Autodesk Fusion 360 part; units mm, degrees
(part 17 of 18)
  spline S9 degree 5 poles (6.448875, 0.349392) (6.446894, 0.350948) (6.442931, 0.354057) (6.436987, 0.358705) (6.429063, 0.364874) (6.419158, 0.372539) (6.409254, 0.380155) (6.399351, 0.387725) (6.389449, 0.395247) (6.379548, 0.402722) (6.369649, 0.410149) (6.359751, 0.417529) (6.349856, 0.424862) (6.339962, 0.432147) (6.330071, 0.439384) (6.320183, 0.446575) (6.310298, 0.453717) (6.300416, 0.460813) (6.290538, 0.467861) (6.280664, 0.474861) (6.270793, 0.481815) (6.260927, 0.48872) (6.251065, 0.495579) (6.241208, 0.50239) (6.231356, 0.509153) (6.221509, 0.515869) (6.211668, 0.522538) (6.201832, 0.52916) (6.192002, 0.535734) (6.182179, 0.54226) (6.172362, 0.54874) (6.162551, 0.555172) (6.152748, 0.561557) (6.142952, 0.567894) (6.133163, 0.574185) (6.123382, 0.580428) (6.113609, 0.586623) (6.103844, 0.592772) (6.094088, 0.598873) (6.084341, 0.604928) (6.074602, 0.610935) (6.064873, 0.616895) (6.055154, 0.622808) (6.045444, 0.628674) (6.035744, 0.634492) (6.026055, 0.640264) (6.016376, 0.645989) (6.006708, 0.651667) (5.997052, 0.657298) (5.987406, 0.662882) (5.977773, 0.66842) (5.968151, 0.67391) (5.958542, 0.679354) (5.948945, 0.684751) (5.93936, 0.690101) (5.929789, 0.695405) (5.920232, 0.700662) (5.910687, 0.705873) (5.901157, 0.711037) (5.891641, 0.716155) (5.882139, 0.721226) (5.872652, 0.726251) (5.86318, 0.73123) (5.853723, 0.736162) (5.844282, 0.741048) (5.834857, 0.745888) (5.825447, 0.750682) (5.816054, 0.75543) (5.806678, 0.760132) (5.797319, 0.764788) (5.787977, 0.769398) (5.778653, 0.773962) (5.769346, 0.778481) (5.760058, 0.782954) (5.750788, 0.787381) (5.741537, 0.791763) (5.732305, 0.7961) (5.723092, 0.800391) (5.713899, 0.804636) (5.704726, 0.808837) (5.695573, 0.812992) (5.686441, 0.817103) (5.677329, 0.821168) (5.668238, 0.825188) (5.659169, 0.829164) (5.650122, 0.833095) (5.641097, 0.836981) (5.632094, 0.840823) (5.623114, 0.84462) (5.614157, 0.848373) (5.605223, 0.852081) (5.596312, 0.855745) (5.587426, 0.859365) (5.578564, 0.862942) (5.569726, 0.866474) (5.560914, 0.869962) (5.552126, 0.873407) (5.543364, 0.876808) (5.534628, 0.880166) (5.525918, 0.88348) (5.517235, 0.886752) (5.508578, 0.88998) (5.499949, 0.893164) (5.491347, 0.896307) (5.482773, 0.899406) (5.474226, 0.902462) (5.465709, 0.905476) (5.45722, 0.908448) (5.448761, 0.911377) (5.44033, 0.914264) (5.43193, 0.917109) (5.42356, 0.919913) (5.41522, 0.922674) (5.406911, 0.925394) (5.398634, 0.928072) (5.390388, 0.930709) (5.382174, 0.933305) (5.373992, 0.93586) (5.365842, 0.938374) (5.357726, 0.940847) (5.349643, 0.943279) (5.341593, 0.945672) (5.333578, 0.948023) (5.325597, 0.950335) (5.317651, 0.952607) (5.30974, 0.954839) (5.301864, 0.957031) (5.294024, 0.959184) (5.28622, 0.961298) (5.278453, 0.963372) (5.270723, 0.965408) (5.263031, 0.967405) (5.255375, 0.969364) (5.247758, 0.971284) (5.24018, 0.973166) (5.23264, 0.97501) (5.22514, 0.976816) (5.217679, 0.978584) (5.210258, 0.980316) (5.202878, 0.98201) (5.195538, 0.983667) (5.18824, 0.985287) (5.180983, 0.986871) (5.173768, 0.988419) (5.166596, 0.98993) (5.159466, 0.991406) (5.152379, 0.992846) (5.145336, 0.994251) (5.138338, 0.99562) (5.131383, 0.996955) (5.124474, 0.998254) (5.117609, 0.99952) (5.110791, 1.000751) (5.104018, 1.001948) (5.097292, 1.003112) (5.090613, 1.004242) (5.083981, 1.005339) (5.077397, 1.006403) (5.070862, 1.007435) (5.064375, 1.008434) (5.057937, 1.009401) (5.051549, 1.010337) (5.045211, 1.011241) (5.038924, 1.012114) (5.032687, 1.012955) (5.026502, 1.013767) (5.020368, 1.014548) (5.014287, 1.015299) (5.008259, 1.01602) (5.002284, 1.016712) (4.996363, 1.017375) (4.990496, 1.01801) (4.984684, 1.018616) (4.978927, 1.019194) (4.973225, 1.019744) (4.96758, 1.020267) (4.961991, 1.020763) (4.95646, 1.021233) (4.950986, 1.021676) (4.945571, 1.022094) (4.940214, 1.022486) (4.934916, 1.022853) (4.929678, 1.023195) (4.9245, 1.023513) (4.919383, 1.023807) (4.914327, 1.024078) (4.909334, 1.024325) (4.904402, 1.02455) (4.899534, 1.024753) (4.894729, 1.024934) (4.889988, 1.025093) (4.885311, 1.025232) (4.8807, 1.025351) (4.876155, 1.025449) (4.871676, 1.025528) (4.867264, 1.025588) (4.862919, 1.025629) (4.858642, 1.025653) (4.854434, 1.025658) (4.850296, 1.025647) (4.846227, 1.02562) (4.842229, 1.025576) (4.838302, 1.025517) (4.834447, 1.025444) (4.830665, 1.025356) (4.826955, 1.025254) (4.82332, 1.025139) (4.819758, 1.025012) (4.816272, 1.024872) (4.812862, 1.024722) (4.809528, 1.024561) (4.806271, 1.024389) (4.803092, 1.024208) (4.799992, 1.024019) (4.796971, 1.023821) (4.79403, 1.023616) (4.79117, 1.023404) (4.788391, 1.023186) (4.785695, 1.022963) (4.783081, 1.022736) (4.780552, 1.022504) (4.778107, 1.02227) (4.775748, 1.022033) (4.773475, 1.021795) (4.771289, 1.021556) (4.769192, 1.021318) (4.767183, 1.02108) (4.765263, 1.020844) (4.763435, 1.020612) (4.761697, 1.020383) (4.760053, 1.020158) (4.758501, 1.019939) (4.757044, 1.019727) (4.755682, 1.019523) (4.754417, 1.019326) (4.753248, 1.019139) (4.752177, 1.018962) (4.751206, 1.018798) (4.750336, 1.018647) (4.749568, 1.01851) (4.748903, 1.018389) (4.748453, 1.018304) (4.748162, 1.018248) (4.747988, 1.018213) (4.747907, 1.018197) knots -1 -1 -1 -1 -1 -1 -0.99583333 -0.99166667 -0.9875 -0.98333333 -0.97916667 -0.975 -0.97083333 -0.96666667 -0.9625 -0.95833333 -0.95416667 -0.95 -0.94583333 -0.94166667 -0.9375 -0.93333333 -0.92916667 -0.925 -0.92083333 -0.91666667 -0.9125 -0.90833333 -0.90416667 -0.9 -0.89583333 -0.89166667 -0.8875 -0.88333333 -0.87916667 -0.875 -0.87083333 -0.86666667 -0.8625 -0.85833333 -0.85416667 -0.85 -0.84583333 -0.84166667 -0.8375 -0.83333333 -0.82916667 -0.825 -0.82083333 -0.81666667 -0.8125 -0.80833333 -0.80416667 -0.8 -0.79583333 -0.79166667 -0.7875 -0.78333333 -0.77916667 -0.775 -0.77083333 -0.76666667 -0.7625 -0.75833333 -0.75416667 -0.75 -0.74583333 -0.74166667 -0.7375 -0.73333333 -0.72916667 -0.725 -0.72083333 -0.71666667 -0.7125 -0.70833333 -0.70416667 -0.7 -0.69583333 -0.69166667 -0.6875 -0.68333333 -0.67916667 -0.675 -0.67083333 -0.66666667 -0.6625 -0.65833333 -0.65416667 -0.65 -0.64583333 -0.64166667 -0.6375 -0.63333333 -0.62916667 -0.625 -0.62083333 -0.61666667 -0.6125 -0.60833333 -0.60416667 -0.6 -0.59583333 -0.59166667 -0.5875 -0.58333333 -0.57916667 -0.575 -0.57083333 -0.56666667 -0.5625 -0.55833333 -0.55416667 -0.55 -0.54583333 -0.54166667 -0.5375 -0.53333333 -0.52916667 -0.525 -0.52083333 -0.51666667 -0.5125 -0.50833333 -0.50416667 -0.5 -0.49583333 -0.49166667 -0.4875 -0.48333333 -0.47916667 -0.475 -0.47083333 -0.46666667 -0.4625 -0.45833333 -0.45416667 -0.45 -0.44583333 -0.44166667 -0.4375 -0.43333333 -0.42916667 -0.425 -0.42083333 -0.41666667 -0.4125 -0.40833333 -0.40416667 -0.4 -0.39583333 -0.39166667 -0.3875 -0.38333333 -0.37916667 -0.375 -0.37083333 -0.36666667 -0.3625 -0.35833333 -0.35416667 -0.35 -0.34583333 -0.34166667 -0.3375 -0.33333333 -0.32916667 -0.325 -0.32083333 -0.31666667 -0.3125 -0.30833333 -0.30416667 -0.3 -0.29583333 -0.29166667 -0.2875 -0.28333333 -0.27916667 -0.275 -0.27083333 -0.26666667 -0.2625 -0.25833333 -0.25416667 -0.25 -0.24583333 -0.24166667 -0.2375 -0.23333333 -0.22916667 -0.225 -0.22083333 -0.21666667 -0.2125 -0.20833333 -0.20416667 -0.2 -0.19583333 -0.19166667 -0.1875 -0.18333333 -0.17916667 -0.175 -0.17083333 -0.16666667 -0.1625 -0.15833333 -0.15416667 -0.15 -0.14583333 -0.14166667 -0.1375 -0.13333333 -0.12916667 -0.125 -0.12083333 -0.11666667 -0.1125 -0.10833333 -0.10416667 -0.1 -0.09583333 -0.09166667 -0.0875 -0.08333333 -0.07916667 -0.075 -0.07083333 -0.06666667 -0.0625 -0.05833333 -0.05416667 -0.05 -0.04583333 -0.04166667 -0.0375 -0.03333333 -0.02916667 -0.025 -0.02083333 -0.01666667 -0.0125 -0.00833333 -0.00416667 0 0 0 0 0 0
  line L18 (4.747907, 1.018197) -> (4.747144, 1.018043)
  line L19 (4.747144, 1.018043) -> (3.473116, 0.744823)
  arc A10 (3.473116, 0.744823) -> (2.982533, 1.929195) centre (0, 0) ccw
  line L20 (2.982533, 1.929195) -> (4.076603, 2.636873)
  line L21 (4.076603, 2.636873) -> (4.077251, 2.637303)
  spline S10 degree 5 poles (4.077251, 2.637303) (4.07732, 2.637349) (4.077467, 2.637448) (4.077713, 2.637613) (4.078091, 2.637872) (4.078647, 2.638256) (4.079287, 2.638703) (4.080009, 2.639211) (4.080812, 2.639782) (4.081694, 2.640414) (4.082653, 2.641108) (4.083687, 2.641864) (4.084794, 2.642682) (4.085975, 2.643562) (4.087226, 2.644505) (4.088548, 2.645509) (4.089938, 2.646575) (4.091396, 2.647704) (4.09292, 2.648895) (4.094508, 2.650147) (4.09616, 2.651462) (4.097875, 2.652839) (4.09965, 2.654277) (4.101486, 2.655778) (4.10338, 2.657341) (4.105333, 2.658966) (4.107341, 2.660653) (4.109406, 2.662402) (4.111524, 2.664213) (4.113697, 2.666085) (4.115921, 2.66802) (4.118197, 2.670016) (4.120524, 2.672074) (4.122899, 2.674194) (4.125323, 2.676376) (4.127795, 2.678619) (4.130313, 2.680924) (4.132877, 2.683291) (4.135485, 2.685719) (4.138137, 2.688209) (4.140832, 2.69076) (4.143569, 2.693372) (4.146347, 2.696046) (4.149165, 2.698781) (4.152023, 2.701577) (4.154919, 2.704435) (4.157854, 2.707354) (4.160825, 2.710333) (4.163832, 2.713374) (4.166875, 2.716475) (4.169953, 2.719637) (4.173064, 2.72286) (4.176209, 2.726144) (4.179385, 2.729488) (4.182594, 2.732893) (4.185834, 2.736358) (4.189103, 2.739884) (4.192402, 2.74347) (4.19573, 2.747116) (4.199087, 2.750822) (4.20247, 2.754588) (4.20588, 2.758415) (4.209317, 2.762301) (4.212779, 2.766246) (4.216265, 2.770252) (4.219776, 2.774317) (4.22331, 2.778442) (4.226867, 2.782626) (4.230446, 2.786869) (4.234047, 2.791172) (4.237669, 2.795533) (4.241312, 2.799954) (4.244974, 2.804434) (4.248655, 2.808972) (4.252355, 2.813569) (4.256073, 2.818225) (4.259809, 2.822939) (4.263561, 2.827712) (4.26733, 2.832543) (4.271115, 2.837432) (4.274915, 2.842379) (4.278729, 2.847385) (4.282558, 2.852448) (4.286401, 2.857569) (4.290256, 2.862747) (4.294125, 2.867983) (4.298005, 2.873277) (4.301897, 2.878627) (4.3058, 2.884035) (4.309713, 2.8895) (4.313637, 2.895022) (4.31757, 2.900601) (4.321513, 2.906237) (4.325463, 2.911929) (4.329422, 2.917678) (4.333389, 2.923482) (4.337363, 2.929344) (4.341344, 2.935261) (4.34533, 2.941234) (4.349323, 2.947263) (4.353321, 2.953348) (4.357324, 2.959489) (4.361331, 2.965685) (4.365343, 2.971936) (4.369358, 2.978243) (4.373376, 2.984604) (4.377397, 2.991021) (4.38142, 2.997493) (4.385445, 3.004019) (4.389471, 3.0106) (4.393499, 3.017235) (4.397527, 3.023924) (4.401555, 3.030668) (4.405583, 3.037466) (4.409611, 3.044318) (4.413637, 3.051223) (4.417663, 3.058182) (4.421686, 3.065195) (4.425707, 3.072261) (4.429726, 3.07938) (4.433742, 3.086552) (4.437754, 3.093777) (4.441763, 3.101056) (4.445768, 3.108386) (4.449768, 3.11577) (4.453764, 3.123205) (4.457754, 3.130693) (4.461739, 3.138233) (4.465718, 3.145825) (4.469691, 3.153469) (4.473657, 3.161164) (4.477616, 3.168911) (4.481568, 3.17671) (4.485512, 3.184559) (4.489449, 3.19246) (4.493377, 3.200412) (4.497297, 3.208415) (4.501207, 3.216468) (4.505108, 3.224571) (4.509, 3.232725) (4.512882, 3.24093) (4.516753, 3.249184) (4.520614, 3.257488) (4.524464, 3.265842) (4.528302, 3.274246) (4.532129, 3.282699) (4.535945, 3.291202) (4.539748, 3.299753) (4.543538, 3.308354) (4.547316, 3.317004) (4.551081, 3.325702) (4.554832, 3.334449) (4.55857, 3.343244) (4.562294, 3.352087) (4.566003, 3.360979) (4.569698, 3.369918) (4.573378, 3.378906) (4.577043, 3.387941) (4.580693, 3.397023) (4.584327, 3.406153) (4.587945, 3.41533) (4.591546, 3.424554) (4.595131, 3.433824) (4.598699, 3.443142) (4.602251, 3.452506) (4.605784, 3.461916) (4.609301, 3.471373) (4.612799, 3.480876) (4.616279, 3.490424) (4.619741, 3.500019) (4.623184, 3.509659) (4.626608, 3.519344) (4.630013, 3.529075) (4.633399, 3.538851) (4.636764, 3.548671) (4.64011, 3.558537) (4.643436, 3.568447) (4.646741, 3.578402) (4.650026, 3.588401) (4.653289, 3.598444) (4.656532, 3.608531) (4.659752, 3.618662) (4.662952, 3.628837) (4.666129, 3.639055) (4.669284, 3.649317) (4.672417, 3.659621) (4.675527, 3.669969) (4.678615, 3.68036) (4.681679, 3.690793) (4.68472, 3.701269) (4.687737, 3.711787) (4.690731, 3.722347) (4.693701, 3.732949) (4.696647, 3.743594) (4.699568, 3.75428) (4.702464, 3.765007) (4.705336, 3.775776) (4.708182, 3.786586) (4.711004, 3.797437) (4.713799, 3.808329) (4.716569, 3.819262) (4.719314, 3.830235) (4.722032, 3.841249) (4.724723, 3.852302) (4.727389, 3.863396) (4.730027, 3.87453) (4.732638, 3.885704) (4.735223, 3.896917) (4.73778, 3.908169) (4.740309, 3.919461) (4.742811, 3.930791) (4.745285, 3.942161) (4.74773, 3.953569) (4.750148, 3.965016) (4.752536, 3.976501) (4.754896, 3.988024) (4.757228, 3.999586) (4.75953, 4.011185) (4.761803, 4.022822) (4.764046, 4.034497) (4.76626, 4.046208) (4.768444, 4.057958) (4.770598, 4.069744) (4.772721, 4.081567) (4.774815, 4.093426) (4.776878, 4.105322) (4.77891, 4.117255) (4.780911, 4.129223) (4.782881, 4.141228) (4.78482, 4.153268) (4.786728, 4.165345) (4.788604, 4.177456) (4.790449, 4.189603) (4.792261, 4.201786) (4.794041, 4.214003) (4.795789, 4.226254) (4.797505, 4.238541) (4.799187, 4.250862) (4.800837, 4.263216) (4.802455, 4.275606) (4.804039, 4.288029) (4.80528, 4.297995) (4.806196, 4.305485) (4.8068, 4.310485) (4.807101, 4.312986) knots 0 0 0 0 0 0 0.00416667 0.00833333 0.0125 0.01666667 0.02083333 0.025 0.02916667 0.03333333 0.0375 0.04166667 0.04583333 0.05 0.05416667 0.05833333 0.0625 0.06666667 0.07083333 0.075 0.07916667 0.08333333 0.0875 0.09166667 0.09583333 0.1 0.10416667 0.10833333 0.1125 0.11666667 0.12083333 0.125 0.12916667 0.13333333 0.1375 0.14166667 0.14583333 0.15 0.15416667 0.15833333 0.1625 0.16666667 0.17083333 0.175 0.17916667 0.18333333 0.1875 0.19166667 0.19583333 0.2 0.20416667 0.20833333 0.2125 0.21666667 0.22083333 0.225 0.22916667 0.23333333 0.2375 0.24166667 0.24583333 0.25 0.25416667 0.25833333 0.2625 0.26666667 0.27083333 0.275 0.27916667 0.28333333 0.2875 0.29166667 0.29583333 0.3 0.30416667 0.30833333 0.3125 0.31666667 0.32083333 0.325 0.32916667 0.33333333 0.3375 0.34166667 0.34583333 0.35 0.35416667 0.35833333 0.3625 0.36666667 0.37083333 0.375 0.37916667 0.38333333 0.3875 0.39166667 0.39583333 0.4 0.40416667 0.40833333 0.4125 0.41666667 0.42083333 0.425 0.42916667 0.43333333 0.4375 0.44166667 0.44583333 0.45 0.45416667 0.45833333 0.4625 0.46666667 0.47083333 0.475 0.47916667 0.48333333 0.4875 0.49166667 0.49583333 0.5 0.50416667 0.50833333 0.5125 0.51666667 0.52083333 0.525 0.52916667 0.53333333 0.5375 0.54166667 0.54583333 0.55 0.55416667 0.55833333 0.5625 0.56666667 0.57083333 0.575 0.57916667 0.58333333 0.5875 0.59166667 0.59583333 0.6 0.60416667 0.60833333 0.6125 0.61666667 0.62083333 0.625 0.62916667 0.63333333 0.6375 0.64166667 0.64583333 0.65 0.65416667 0.65833333 0.6625 0.66666667 0.67083333 0.675 0.67916667 0.68333333 0.6875 0.69166667 0.69583333 0.7 0.70416667 0.70833333 0.7125 0.71666667 0.72083333 0.725 0.72916667 0.73333333 0.7375 0.74166667 0.74583333 0.75 0.75416667 0.75833333 0.7625 0.76666667 0.77083333 0.775 0.77916667 0.78333333 0.7875 0.79166667 0.79583333 0.8 0.80416667 0.80833333 0.8125 0.81666667 0.82083333 0.825 0.82916667 0.83333333 0.8375 0.84166667 0.84583333 0.85 0.85416667 0.85833333 0.8625 0.86666667 0.87083333 0.875 0.87916667 0.88333333 0.8875 0.89166667 0.89583333 0.9 0.90416667 0.90833333 0.9125 0.91666667 0.92083333 0.925 0.92916667 0.93333333 0.9375 0.94166667 0.94583333 0.95 0.95416667 0.95833333 0.9625 0.96666667 0.97083333 0.975 0.97916667 0.98333333 0.9875 0.99166667 0.99583333 1 1 1 1 1 1
  arc A11 (4.807101, 4.312986) -> (4.312986, 4.807101) centre (0, 0) ccw
  spline S11 degree 5 poles (4.312986, 4.807101) (4.310485, 4.8068) (4.305485, 4.806196) (4.297995, 4.80528) (4.288029, 4.804039) (4.275606, 4.802455) (4.263216, 4.800837) (4.250862, 4.799187) (4.238541, 4.797505) (4.226254, 4.795789) (4.214003, 4.794041) (4.201786, 4.792261) (4.189603, 4.790449) (4.177456, 4.788604) (4.165345, 4.786728) (4.153268, 4.78482) (4.141228, 4.782881) (4.129223, 4.780911) (4.117255, 4.77891) (4.105322, 4.776878) (4.093426, 4.774815) (4.081567, 4.772721) (4.069744, 4.770598) (4.057958, 4.768444) (4.046208, 4.76626) (4.034497, 4.764046) (4.022822, 4.761803) (4.011185, 4.75953) (3.999586, 4.757228) (3.988024, 4.754896) (3.976501, 4.752536) (3.965016, 4.750148) (3.953569, 4.74773) (3.942161, 4.745285) (3.930791, 4.742811) (3.919461, 4.740309) (3.908169, 4.73778) (3.896917, 4.735223) (3.885704, 4.732638) (3.87453, 4.730027) (3.863396, 4.727389) (3.852302, 4.724723) (3.841249, 4.722032) (3.830235, 4.719314) (3.819262, 4.716569) (3.808329, 4.713799) (3.797437, 4.711004) (3.786586, 4.708182) (3.775776, 4.705336) (3.765007, 4.702464) (3.75428, 4.699568) (3.743594, 4.696647) (3.732949, 4.693701) (3.722347, 4.690731) (3.711787, 4.687737) (3.701269, 4.68472) (3.690793, 4.681679) (3.68036, 4.678615) (3.669969, 4.675527) (3.659621, 4.672417) (3.649317, 4.669284) (3.639055, 4.666129) (3.628837, 4.662952) (3.618662, 4.659752) (3.608531, 4.656532) (3.598444, 4.653289) (3.588401, 4.650026) (3.578402, 4.646741) (3.568447, 4.643436) (3.558537, 4.64011) (3.548671, 4.636764) (3.538851, 4.633399) (3.529075, 4.630013) (3.519344, 4.626608) (3.509659, 4.623184) (3.500019, 4.619741) (3.490424, 4.616279) (3.480876, 4.612799) (3.471373, 4.609301) (3.461916, 4.605784) (3.452506, 4.602251) (3.443142, 4.598699) (3.433824, 4.595131) (3.424554, 4.591546) (3.41533, 4.587945) (3.406153, 4.584327) (3.397023, 4.580693) (3.387941, 4.577043) (3.378906, 4.573378) (3.369918, 4.569698) (3.360979, 4.566003) (3.352087, 4.562294) (3.343244, 4.55857) (3.334449, 4.554832) (3.325702, 4.551081) (3.317004, 4.547316) (3.308354, 4.543538) (3.299753, 4.539748) (3.291202, 4.535945) (3.282699, 4.532129) (3.274246, 4.528302) (3.265842, 4.524464) (3.257488, 4.520614) (3.249184, 4.516753) (3.24093, 4.512882) (3.232725, 4.509) (3.224571, 4.505108) (3.216468, 4.501207) (3.208415, 4.497297) (3.200412, 4.493377) (3.19246, 4.489449) (3.184559, 4.485512) (3.17671, 4.481568) (3.168911, 4.477616) (3.161164, 4.473657) (3.153469, 4.469691) (3.145825, 4.465718) (3.138233, 4.461739) (3.130693, 4.457754) (3.123205, 4.453764) (3.11577, 4.449768) (3.108386, 4.445768) (3.101056, 4.441763) (3.093777, 4.437754) (3.086552, 4.433742) (3.07938, 4.429726) (3.072261, 4.425707) (3.065195, 4.421686) (3.058182, 4.417663) (3.051223, 4.413637) (3.044318, 4.409611) (3.037466, 4.405583) (3.030668, 4.401555) (3.023924, 4.397527) (3.017235, 4.393499) (3.0106, 4.389471) (3.004019, 4.385445) (2.997493, 4.38142) (2.991021, 4.377397) (2.984604, 4.373376) (2.978243, 4.369358) (2.971936, 4.365343) (2.965685, 4.361331) (2.959489, 4.357324) (2.953348, 4.353321) (2.947263, 4.349323) (2.941234, 4.34533) (2.935261, 4.341344) (2.929344, 4.337363) (2.923482, 4.333389) (2.917678, 4.329422) (2.911929, 4.325463) (2.906237, 4.321513) (2.900601, 4.31757) (2.895022, 4.313637) (2.8895, 4.309713) (2.884035, 4.3058) (2.878627, 4.301897) (2.873277, 4.298005) (2.867983, 4.294125) (2.862747, 4.290256) (2.857569, 4.286401) (2.852448, 4.282558) (2.847385, 4.278729) (2.842379, 4.274915) (2.837432, 4.271115) (2.832543, 4.26733) (2.827712, 4.263561) (2.822939, 4.259809) (2.818225, 4.256073) (2.813569, 4.252355) (2.808972, 4.248655) (2.804434, 4.244974) (2.799954, 4.241312) (2.795533, 4.237669) (2.791172, 4.234047) (2.786869, 4.230446) (2.782626, 4.226867) (2.778442, 4.22331) (2.774317, 4.219776) (2.770252, 4.216265) (2.766246, 4.212779) (2.762301, 4.209317) (2.758415, 4.20588) (2.754588, 4.20247) (2.750822, 4.199087) (2.747116, 4.19573) (2.74347, 4.192402) (2.739884, 4.189103) (2.736358, 4.185834) (2.732893, 4.182594) (2.729488, 4.179385) (2.726144, 4.176209) (2.72286, 4.173064) (2.719637, 4.169953) (2.716475, 4.166875) (2.713374, 4.163832) (2.710333, 4.160825) (2.707354, 4.157854) (2.704435, 4.154919) (2.701577, 4.152023) (2.698781, 4.149165) (2.696046, 4.146347) (2.693372, 4.143569) (2.69076, 4.140832) (2.688209, 4.138137) (2.685719, 4.135485) (2.683291, 4.132877) (2.680924, 4.130313) (2.678619, 4.127795) (2.676376, 4.125323) (2.674194, 4.122899) (2.672074, 4.120524) (2.670016, 4.118197) (2.66802, 4.115921) (2.666085, 4.113697) (2.664213, 4.111524) (2.662402, 4.109406) (2.660653, 4.107341) (2.658966, 4.105333) (2.657341, 4.10338) (2.655778, 4.101486) (2.654277, 4.09965) (2.652839, 4.097875) (2.651462, 4.09616) (2.650147, 4.094508) (2.648895, 4.09292) (2.647704, 4.091396) (2.646575, 4.089938) (2.645509, 4.088548) (2.644505, 4.087226) (2.643562, 4.085975) (2.642682, 4.084794) (2.641864, 4.083687) (2.641108, 4.082653) (2.640414, 4.081694) (2.639782, 4.080812) (2.639211, 4.080009) (2.638703, 4.079287) (2.638256, 4.078647) (2.637872, 4.078091) (2.637613, 4.077713) (2.637448, 4.077467) (2.637349, 4.07732) (2.637303, 4.077251) knots -1 -1 -1 -1 -1 -1 -0.99583333 -0.99166667 -0.9875 -0.98333333 -0.97916667 -0.975 -0.97083333 -0.96666667 -0.9625 -0.95833333 -0.95416667 -0.95 -0.94583333 -0.94166667 -0.9375 -0.93333333 -0.92916667 -0.925 -0.92083333 -0.91666667 -0.9125 -0.90833333 -0.90416667 -0.9 -0.89583333 -0.89166667 -0.8875 -0.88333333 -0.87916667 -0.875 -0.87083333 -0.86666667 -0.8625 -0.85833333 -0.85416667 -0.85 -0.84583333 -0.84166667 -0.8375 -0.83333333 -0.82916667 -0.825 -0.82083333 -0.81666667 -0.8125 -0.80833333 -0.80416667 -0.8 -0.79583333 -0.79166667 -0.7875 -0.78333333 -0.77916667 -0.775 -0.77083333 -0.76666667 -0.7625 -0.75833333 -0.75416667 -0.75 -0.74583333 -0.74166667 -0.7375 -0.73333333 -0.72916667 -0.725 -0.72083333 -0.71666667 -0.7125 -0.70833333 -0.70416667 -0.7 -0.69583333 -0.69166667 -0.6875 -0.68333333 -0.67916667 -0.675 -0.67083333 -0.66666667 -0.6625 -0.65833333 -0.65416667 -0.65 -0.64583333 -0.64166667 -0.6375 -0.63333333 -0.62916667 -0.625 -0.62083333 -0.61666667 -0.6125 -0.60833333 -0.60416667 -0.6 -0.59583333 -0.59166667 -0.5875 -0.58333333 -0.57916667 -0.575 -0.57083333 -0.56666667 -0.5625 -0.55833333 -0.55416667 -0.55 -0.54583333 -0.54166667 -0.5375 -0.53333333 -0.52916667 -0.525 -0.52083333 -0.51666667 -0.5125 -0.50833333 -0.50416667 -0.5 -0.49583333 -0.49166667 -0.4875 -0.48333333 -0.47916667 -0.475 -0.47083333 -0.46666667 -0.4625 -0.45833333 -0.45416667 -0.45 -0.44583333 -0.44166667 -0.4375 -0.43333333 -0.42916667 -0.425 -0.42083333 -0.41666667 -0.4125 -0.40833333 -0.40416667 -0.4 -0.39583333 -0.39166667 -0.3875 -0.38333333 -0.37916667 -0.375 -0.37083333 -0.36666667 -0.3625 -0.35833333 -0.35416667 -0.35 -0.34583333 -0.34166667 -0.3375 -0.33333333 -0.32916667 -0.325 -0.32083333 -0.31666667 -0.3125 -0.30833333 -0.30416667 -0.3 -0.29583333 -0.29166667 -0.2875 -0.28333333 -0.27916667 -0.275 -0.27083333 -0.26666667 -0.2625 -0.25833333 -0.25416667 -0.25 -0.24583333 -0.24166667 -0.2375 -0.23333333 -0.22916667 -0.225 -0.22083333 -0.21666667 -0.2125 -0.20833333 -0.20416667 -0.2 -0.19583333 -0.19166667 -0.1875 -0.18333333 -0.17916667 -0.175 -0.17083333 -0.16666667 -0.1625 -0.15833333 -0.15416667 -0.15 -0.14583333 -0.14166667 -0.1375 -0.13333333 -0.12916667 -0.125 -0.12083333 -0.11666667 -0.1125 -0.10833333 -0.10416667 -0.1 -0.09583333 -0.09166667 -0.0875 -0.08333333 -0.07916667 -0.075 -0.07083333 -0.06666667 -0.0625 -0.05833333 -0.05416667 -0.05 -0.04583333 -0.04166667 -0.0375 -0.03333333 -0.02916667 -0.025 -0.02083333 -0.01666667 -0.0125 -0.00833333 -0.00416667 0 0 0 0 0 0
  line L22 (2.637303, 4.077251) -> (2.636873, 4.076603)
  line L23 (2.636873, 4.076603) -> (1.929195, 2.982533)
  arc A12 (1.929195, 2.982533) -> (0.744823, 3.473116) centre (0, 0) ccw
  line L24 (0.744823, 3.473116) -> (1.018043, 4.747144)
  line L25 (1.018043, 4.747144) -> (1.018197, 4.747907)
  spline S12 degree 5 poles (1.018197, 4.747907) (1.018213, 4.747988) (1.018248, 4.748162) (1.018304, 4.748453) (1.018389, 4.748903) (1.01851, 4.749568) (1.018647, 4.750336) (1.018798, 4.751206) (1.018962, 4.752177) (1.019139, 4.753248) (1.019326, 4.754417) (1.019523, 4.755682) (1.019727, 4.757044) (1.019939, 4.758501) (1.020158, 4.760053) (1.020383, 4.761697) (1.020612, 4.763435) (1.020844, 4.765263) (1.02108, 4.767183) (1.021318, 4.769192) (1.021556, 4.771289) (1.021795, 4.773475) (1.022033, 4.775748) (1.02227, 4.778107) (1.022504, 4.780552) (1.022736, 4.783081) (1.022963, 4.785695) (1.023186, 4.788391) (1.023404, 4.79117) (1.023616, 4.79403) (1.023821, 4.796971) (1.024019, 4.799992) (1.024208, 4.803092) (1.024389, 4.806271) (1.024561, 4.809528) (1.024722, 4.812862) (1.024872, 4.816272) (1.025012, 4.819758) (1.025139, 4.82332) (1.025254, 4.826955) (1.025356, 4.830665) (1.025444, 4.834447) (1.025517, 4.838302) (1.025576, 4.842229) (1.02562, 4.846227) (1.025647, 4.850296) (1.025658, 4.854434) (1.025653, 4.858642) (1.025629, 4.862919) (1.025588, 4.867264) (1.025528, 4.871676) (1.025449, 4.876155) (1.025351, 4.8807) (1.025232, 4.885311) (1.025093, 4.889988) (1.024934, 4.894729) (1.024753, 4.899534) (1.02455, 4.904402) (1.024325, 4.909334) (1.024078, 4.914327) (1.023807, 4.919383) (1.023513, 4.9245) (1.023195, 4.929678) (1.022853, 4.934916) (1.022486, 4.940214) (1.022094, 4.945571) (1.021676, 4.950986) (1.021233, 4.95646) (1.020763, 4.961991) (1.020267, 4.96758) (1.019744, 4.973225) (1.019194, 4.978927) (1.018616, 4.984684) (1.01801, 4.990496) (1.017375, 4.996363) (1.016712, 5.002284) (1.01602, 5.008259) (1.015299, 5.014287) (1.014548, 5.020368) (1.013767, 5.026502) (1.012955, 5.032687) (1.012114, 5.038924) (1.011241, 5.045211) (1.010337, 5.051549) (1.009401, 5.057937) (1.008434, 5.064375) (1.007435, 5.070862) (1.006403, 5.077397) (1.005339, 5.083981) (1.004242, 5.090613) (1.003112, 5.097292) (1.001948, 5.104018) (1.000751, 5.110791) (0.99952, 5.117609) (0.998254, 5.124474) (0.996955, 5.131383) (0.99562, 5.138338) (0.994251, 5.145336) (0.992846, 5.152379) (0.991406, 5.159466) (0.98993, 5.166596) (0.988419, 5.173768) (0.986871, 5.180983) (0.985287, 5.18824) (0.983667, 5.195538) (0.98201, 5.202878) (0.980316, 5.210258) (0.978584, 5.217679) (0.976816, 5.22514) (0.97501, 5.23264) (0.973166, 5.24018) (0.971284, 5.247758) (0.969364, 5.255375) (0.967405, 5.263031) (0.965408, 5.270723) (0.963372, 5.278453) (0.961298, 5.28622) (0.959184, 5.294024) (0.957031, 5.301864) (0.954839, 5.30974) (0.952607, 5.317651) (0.950335, 5.325597) (0.948023, 5.333578) (0.945672, 5.341593) (0.943279, 5.349643) (0.940847, 5.357726) (0.938374, 5.365842) (0.93586, 5.373992) (0.933305, 5.382174) (0.930709, 5.390388) (0.928072, 5.398634) (0.925394, 5.406911) (0.922674, 5.41522) (0.919913, 5.42356) (0.917109, 5.43193) (0.914264, 5.44033) (0.911377, 5.448761) (0.908448, 5.45722) (0.905476, 5.465709) (0.902462, 5.474226) (0.899406, 5.482773) (0.896307, 5.491347) (0.893164, 5.499949) (0.88998, 5.508578) (0.886752, 5.517235) (0.88348, 5.525918) (0.880166, 5.534628) (0.876808, 5.543364) (0.873407, 5.552126) (0.869962, 5.560914) (0.866474, 5.569726) (0.862942, 5.578564) (0.859365, 5.587426) (0.855745, 5.596312) (0.852081, 5.605223) (0.848373, 5.614157) (0.84462, 5.623114) (0.840823, 5.632094) (0.836981, 5.641097) (0.833095, 5.650122) (0.829164, 5.659169) (0.825188, 5.668238) (0.821168, 5.677329) (0.817103, 5.686441) (0.812992, 5.695573) (0.808837, 5.704726) (0.804636, 5.713899) (0.800391, 5.723092) (0.7961, 5.732305) (0.791763, 5.741537) (0.787381, 5.750788) (0.782954, 5.760058) (0.778481, 5.769346) (0.773962, 5.778653) (0.769398, 5.787977) (0.764788, 5.797319) (0.760132, 5.806678) (0.75543, 5.816054) (0.750682, 5.825447) (0.745888, 5.834857) (0.741048, 5.844282) (0.736162, 5.853723) (0.73123, 5.86318) (0.726251, 5.872652) (0.721226, 5.882139) (0.716155, 5.891641) (0.711037, 5.901157) (0.705873, 5.910687) (0.700662, 5.920232) (0.695405, 5.929789) (0.690101, 5.93936) (0.684751, 5.948945) (0.679354, 5.958542) (0.67391, 5.968151) (0.66842, 5.977773) (0.662882, 5.987406) (0.657298, 5.997052) (0.651667, 6.006708) (0.645989, 6.016376) (0.640264, 6.026055) (0.634492, 6.035744) (0.628674, 6.045444) (0.622808, 6.055154) (0.616895, 6.064873) (0.610935, 6.074602) (0.604928, 6.084341) (0.598873, 6.094088) (0.592772, 6.103844) (0.586623, 6.113609) (0.580428, 6.123382) (0.574185, 6.133163) (0.567894, 6.142952) (0.561557, 6.152748) (0.555172, 6.162551) (0.54874, 6.172362) (0.54226, 6.182179) (0.535734, 6.192002) (0.52916, 6.201832) (0.522538, 6.211668) (0.515869, 6.221509) (0.509153, 6.231356) (0.50239, 6.241208) (0.495579, 6.251065) (0.48872, 6.260927) (0.481815, 6.270793) (0.474861, 6.280664) (0.467861, 6.290538) (0.460813, 6.300416) (0.453717, 6.310298) (0.446575, 6.320183) (0.439384, 6.330071) (0.432147, 6.339962) (0.424862, 6.349856) (0.417529, 6.359751) (0.410149, 6.369649) (0.402722, 6.379548) (0.395247, 6.389449) (0.387725, 6.399351) (0.380155, 6.409254) (0.372539, 6.419158) (0.364874, 6.429063) (0.358705, 6.436987) (0.354057, 6.442931) (0.350948, 6.446894) (0.349392, 6.448875) knots 0 0 0 0 0 0 0.00416667 0.00833333 0.0125 0.01666667 0.02083333 0.025 0.02916667 0.03333333 0.0375 0.04166667 0.04583333 0.05 0.05416667 0.05833333 0.0625 0.06666667 0.07083333 0.075 0.07916667 0.08333333 0.0875 0.09166667 0.09583333 0.1 0.10416667 0.10833333 0.1125 0.11666667 0.12083333 0.125 0.12916667 0.13333333 0.1375 0.14166667 0.14583333 0.15 0.15416667 0.15833333 0.1625 0.16666667 0.17083333 0.175 0.17916667 0.18333333 0.1875 0.19166667 0.19583333 0.2 0.20416667 0.20833333 0.2125 0.21666667 0.22083333 0.225 0.22916667 0.23333333 0.2375 0.24166667 0.24583333 0.25 0.25416667 0.25833333 0.2625 0.26666667 0.27083333 0.275 0.27916667 0.28333333 0.2875 0.29166667 0.29583333 0.3 0.30416667 0.30833333 0.3125 0.31666667 0.32083333 0.325 0.32916667 0.33333333 0.3375 0.34166667 0.34583333 0.35 0.35416667 0.35833333 0.3625 0.36666667 0.37083333 0.375 0.37916667 0.38333333 0.3875 0.39166667 0.39583333 0.4 0.40416667 0.40833333 0.4125 0.41666667 0.42083333 0.425 0.42916667 0.43333333 0.4375 0.44166667 0.44583333 0.45 0.45416667 0.45833333 0.4625 0.46666667 0.47083333 0.475 0.47916667 0.48333333 0.4875 0.49166667 0.49583333 0.5 0.50416667 0.50833333 0.5125 0.51666667 0.52083333 0.525 0.52916667 0.53333333 0.5375 0.54166667 0.54583333 0.55 0.55416667 0.55833333 0.5625 0.56666667 0.57083333 0.575 0.57916667 0.58333333 0.5875 0.59166667 0.59583333 0.6 0.60416667 0.60833333 0.6125 0.61666667 0.62083333 0.625 0.62916667 0.63333333 0.6375 0.64166667 0.64583333 0.65 0.65416667 0.65833333 0.6625 0.66666667 0.67083333 0.675 0.67916667 0.68333333 0.6875 0.69166667 0.69583333 0.7 0.70416667 0.70833333 0.7125 0.71666667 0.72083333 0.725 0.72916667 0.73333333 0.7375 0.74166667 0.74583333 0.75 0.75416667 0.75833333 0.7625 0.76666667 0.77083333 0.775 0.77916667 0.78333333 0.7875 0.79166667 0.79583333 0.8 0.80416667 0.80833333 0.8125 0.81666667 0.82083333 0.825 0.82916667 0.83333333 0.8375 0.84166667 0.84583333 0.85 0.85416667 0.85833333 0.8625 0.86666667 0.87083333 0.875 0.87916667 0.88333333 0.8875 0.89166667 0.89583333 0.9 0.90416667 0.90833333 0.9125 0.91666667 0.92083333 0.925 0.92916667 0.93333333 0.9375 0.94166667 0.94583333 0.95 0.95416667 0.95833333 0.9625 0.96666667 0.97083333 0.975 0.97916667 0.98333333 0.9875 0.99166667 0.99583333 1 1 1 1 1 1
  arc A13 (0.349392, 6.448875) -> (-0.349392, 6.448875) centre (0, 0) ccw
  spline S13 degree 5 poles (-0.349392, 6.448875) (-0.350948, 6.446894) (-0.354057, 6.442931) (-0.358705, 6.436987) (-0.364874, 6.429063) (-0.372539, 6.419158) (-0.380155, 6.409254) (-0.387725, 6.399351) (-0.395247, 6.389449) (-0.402722, 6.379548) (-0.410149, 6.369649) (-0.417529, 6.359751) (-0.424862, 6.349856) (-0.432147, 6.339962) (-0.439384, 6.330071) (-0.446575, 6.320183) (-0.453717, 6.310298) (-0.460813, 6.300416) (-0.467861, 6.290538) (-0.474861, 6.280664) (-0.481815, 6.270793) (-0.48872, 6.260927) (-0.495579, 6.251065) (-0.50239, 6.241208) (-0.509153, 6.231356) (-0.515869, 6.221509) (-0.522538, 6.211668) (-0.52916, 6.201832) (-0.535734, 6.192002) (-0.54226, 6.182179) (-0.54874, 6.172362) (-0.555172, 6.162551) (-0.561557, 6.152748) (-0.567894, 6.142952) (-0.574185, 6.133163) (-0.580428, 6.123382) (-0.586623, 6.113609) (-0.592772, 6.103844) (-0.598873, 6.094088) (-0.604928, 6.084341) (-0.610935, 6.074602) (-0.616895, 6.064873) (-0.622808, 6.055154) (-0.628674, 6.045444) (-0.634492, 6.035744) (-0.640264, 6.026055) (-0.645989, 6.016376) (-0.651667, 6.006708) (-0.657298, 5.997052) (-0.662882, 5.987406) (-0.66842, 5.977773) (-0.67391, 5.968151) (-0.679354, 5.958542) (-0.684751, 5.948945) (-0.690101, 5.93936) (-0.695405, 5.929789) (-0.700662, 5.920232) (-0.705873, 5.910687) (-0.711037, 5.901157) (-0.716155, 5.891641) (-0.721226, 5.882139) (-0.726251, 5.872652) (-0.73123, 5.86318) (-0.736162, 5.853723) (-0.741048, 5.844282) (-0.745888, 5.834857) (-0.750682, 5.825447) (-0.75543, 5.816054) (-0.760132, 5.806678) (-0.764788, 5.797319) (-0.769398, 5.787977) (-0.773962, 5.778653) (-0.778481, 5.769346) (-0.782954, 5.760058) (-0.787381, 5.750788) (-0.791763, 5.741537) (-0.7961, 5.732305) (-0.800391, 5.723092) (-0.804636, 5.713899) (-0.808837, 5.704726) (-0.812992, 5.695573) (-0.817103, 5.686441) (-0.821168, 5.677329) (-0.825188, 5.668238) (-0.829164, 5.659169) (-0.833095, 5.650122) (-0.836981, 5.641097) (-0.840823, 5.632094) (-0.84462, 5.623114) (-0.848373, 5.614157) (-0.852081, 5.605223) (-0.855745, 5.596312) (-0.859365, 5.587426) (-0.862942, 5.578564) (-0.866474, 5.569726) (-0.869962, 5.560914) (-0.873407, 5.552126) (-0.876808, 5.543364) (-0.880166, 5.534628) (-0.88348, 5.525918) (-0.886752, 5.517235) (-0.88998, 5.508578) (-0.893164, 5.499949) (-0.896307, 5.491347) (-0.899406, 5.482773) (-0.902462, 5.474226) (-0.905476, 5.465709) (-0.908448, 5.45722) (-0.911377, 5.448761) (-0.914264, 5.44033) (-0.917109, 5.43193) (-0.919913, 5.42356) (-0.922674, 5.41522) (-0.925394, 5.406911) (-0.928072, 5.398634) (-0.930709, 5.390388) (-0.933305, 5.382174) (-0.93586, 5.373992) (-0.938374, 5.365842) (-0.940847, 5.357726) (-0.943279, 5.349643) (-0.945672, 5.341593) (-0.948023, 5.333578) (-0.950335, 5.325597) (-0.952607, 5.317651) (-0.954839, 5.30974) (-0.957031, 5.301864) (-0.959184, 5.294024) (-0.961298, 5.28622) (-0.963372, 5.278453) (-0.965408, 5.270723) (-0.967405, 5.263031) (-0.969364, 5.255375) (-0.971284, 5.247758) (-0.973166, 5.24018) (-0.97501, 5.23264) (-0.976816, 5.22514) (-0.978584, 5.217679) (-0.980316, 5.210258) (-0.98201, 5.202878) (-0.983667, 5.195538) (-0.985287, 5.18824) (-0.986871, 5.180983) (-0.988419, 5.173768) (-0.98993, 5.166596) (-0.991406, 5.159466) (-0.992846, 5.152379) (-0.994251, 5.145336) (-0.99562, 5.138338) (-0.996955, 5.131383) (-0.998254, 5.124474) (-0.99952, 5.117609) (-1.000751, 5.110791) (-1.001948, 5.104018) (-1.003112, 5.097292) (-1.004242, 5.090613) (-1.005339, 5.083981) (-1.006403, 5.077397) (-1.007435, 5.070862) (-1.008434, 5.064375) (-1.009401, 5.057937) (-1.010337, 5.051549) (-1.011241, 5.045211) (-1.012114, 5.038924) (-1.012955, 5.032687) (-1.013767, 5.026502) (-1.014548, 5.020368) (-1.015299, 5.014287) (-1.01602, 5.008259) (-1.016712, 5.002284) (-1.017375, 4.996363) (-1.01801, 4.990496) (-1.018616, 4.984684) (-1.019194, 4.978927) (-1.019744, 4.973225) (-1.020267, 4.96758) (-1.020763, 4.961991) (-1.021233, 4.95646) (-1.021676, 4.950986) (-1.022094, 4.945571) (-1.022486, 4.940214) (-1.022853, 4.934916) (-1.023195, 4.929678) (-1.023513, 4.9245) (-1.023807, 4.919383) (-1.024078, 4.914327) (-1.024325, 4.909334) (-1.02455, 4.904402) (-1.024753, 4.899534) (-1.024934, 4.894729) (-1.025093, 4.889988) (-1.025232, 4.885311) (-1.025351, 4.8807) (-1.025449, 4.876155) (-1.025528, 4.871676) (-1.025588, 4.867264) (-1.025629, 4.862919) (-1.025653, 4.858642) (-1.025658, 4.854434) (-1.025647, 4.850296) (-1.02562, 4.846227) (-1.025576, 4.842229) (-1.025517, 4.838302) (-1.025444, 4.834447) (-1.025356, 4.830665) (-1.025254, 4.826955) (-1.025139, 4.82332) (-1.025012, 4.819758) (-1.024872, 4.816272) (-1.024722, 4.812862) (-1.024561, 4.809528) (-1.024389, 4.806271) (-1.024208, 4.803092) (-1.024019, 4.799992) (-1.023821, 4.796971) (-1.023616, 4.79403) (-1.023404, 4.79117) (-1.023186, 4.788391) (-1.022963, 4.785695) (-1.022736, 4.783081) (-1.022504, 4.780552) (-1.02227, 4.778107) (-1.022033, 4.775748) (-1.021795, 4.773475) (-1.021556, 4.771289) (-1.021318, 4.769192) (-1.02108, 4.767183) (-1.020844, 4.765263) (-1.020612, 4.763435) (-1.020383, 4.761697) (-1.020158, 4.760053) (-1.019939, 4.758501) (-1.019727, 4.757044) (-1.019523, 4.755682) (-1.019326, 4.754417) (-1.019139, 4.753248) (-1.018962, 4.752177) (-1.018798, 4.751206) (-1.018647, 4.750336) (-1.01851, 4.749568) (-1.018389, 4.748903) (-1.018304, 4.748453) (-1.018248, 4.748162) (-1.018213, 4.747988) (-1.018197, 4.747907) knots -1 -1 -1 -1 -1 -1 -0.99583333 -0.99166667 -0.9875 -0.98333333 -0.97916667 -0.975 -0.97083333 -0.96666667 -0.9625 -0.95833333 -0.95416667 -0.95 -0.94583333 -0.94166667 -0.9375 -0.93333333 -0.92916667 -0.925 -0.92083333 -0.91666667 -0.9125 -0.90833333 -0.90416667 -0.9 -0.89583333 -0.89166667 -0.8875 -0.88333333 -0.87916667 -0.875 -0.87083333 -0.86666667 -0.8625 -0.85833333 -0.85416667 -0.85 -0.84583333 -0.84166667 -0.8375 -0.83333333 -0.82916667 -0.825 -0.82083333 -0.81666667 -0.8125 -0.80833333 -0.80416667 -0.8 -0.79583333 -0.79166667 -0.7875 -0.78333333 -0.77916667 -0.775 -0.77083333 -0.76666667 -0.7625 -0.75833333 -0.75416667 -0.75 -0.74583333 -0.74166667 -0.7375 -0.73333333 -0.72916667 -0.725 -0.72083333 -0.71666667 -0.7125 -0.70833333 -0.70416667 -0.7 -0.69583333 -0.69166667 -0.6875 -0.68333333 -0.67916667 -0.675 -0.67083333 -0.66666667 -0.6625 -0.65833333 -0.65416667 -0.65 -0.64583333 -0.64166667 -0.6375 -0.63333333 -0.62916667 -0.625 -0.62083333 -0.61666667 -0.6125 -0.60833333 -0.60416667 -0.6 -0.59583333 -0.59166667 -0.5875 -0.58333333 -0.57916667 -0.575 -0.57083333 -0.56666667 -0.5625 -0.55833333 -0.55416667 -0.55 -0.54583333 -0.54166667 -0.5375 -0.53333333 -0.52916667 -0.525 -0.52083333 -0.51666667 -0.5125 -0.50833333 -0.50416667 -0.5 -0.49583333 -0.49166667 -0.4875 -0.48333333 -0.47916667 -0.475 -0.47083333 -0.46666667 -0.4625 -0.45833333 -0.45416667 -0.45 -0.44583333 -0.44166667 -0.4375 -0.43333333 -0.42916667 -0.425 -0.42083333 -0.41666667 -0.4125 -0.40833333 -0.40416667 -0.4 -0.39583333 -0.39166667 -0.3875 -0.38333333 -0.37916667 -0.375 -0.37083333 -0.36666667 -0.3625 -0.35833333 -0.35416667 -0.35 -0.34583333 -0.34166667 -0.3375 -0.33333333 -0.32916667 -0.325 -0.32083333 -0.31666667 -0.3125 -0.30833333 -0.30416667 -0.3 -0.29583333 -0.29166667 -0.2875 -0.28333333 -0.27916667 -0.275 -0.27083333 -0.26666667 -0.2625 -0.25833333 -0.25416667 -0.25 -0.24583333 -0.24166667 -0.2375 -0.23333333 -0.22916667 -0.225 -0.22083333 -0.21666667 -0.2125 -0.20833333 -0.20416667 -0.2 -0.19583333 -0.19166667 -0.1875 -0.18333333 -0.17916667 -0.175 -0.17083333 -0.16666667 -0.1625 -0.15833333 -0.15416667 -0.15 -0.14583333 -0.14166667 -0.1375 -0.13333333 -0.12916667 -0.125 -0.12083333 -0.11666667 -0.1125 -0.10833333 -0.10416667 -0.1 -0.09583333 -0.09166667 -0.0875 -0.08333333 -0.07916667 -0.075 -0.07083333 -0.06666667 -0.0625 -0.05833333 -0.05416667 -0.05 -0.04583333 -0.04166667 -0.0375 -0.03333333 -0.02916667 -0.025 -0.02083333 -0.01666667 -0.0125 -0.00833333 -0.00416667 0 0 0 0 0 0
  line L26 (-1.018197, 4.747907) -> (-1.018043, 4.747144)
  line L27 (-1.018043, 4.747144) -> (-0.744823, 3.473116)
  arc A14 (-0.744823, 3.473116) -> (-1.929195, 2.982533) centre (0, 0) ccw
  line L28 (-1.929195, 2.982533) -> (-2.636873, 4.076603)
  line L29 (-2.636873, 4.076603) -> (-2.637303, 4.077251)
  spline S14 degree 5 poles (-2.637303, 4.077251) (-2.637349, 4.07732) (-2.637448, 4.077467) (-2.637613, 4.077713) (-2.637872, 4.078091) (-2.638256, 4.078647) (-2.638703, 4.079287) (-2.639211, 4.080009) (-2.639782, 4.080812) (-2.640414, 4.081694) (-2.641108, 4.082653) (-2.641864, 4.083687) (-2.642682, 4.084794) (-2.643562, 4.085975) (-2.644505, 4.087226) (-2.645509, 4.088548) (-2.646575, 4.089938) (-2.647704, 4.091396) (-2.648895, 4.09292) (-2.650147, 4.094508) (-2.651462, 4.09616) (-2.652839, 4.097875) (-2.654277, 4.09965) (-2.655778, 4.101486) (-2.657341, 4.10338) (-2.658966, 4.105333) (-2.660653, 4.107341) (-2.662402, 4.109406) (-2.664213, 4.111524) (-2.666085, 4.113697) (-2.66802, 4.115921) (-2.670016, 4.118197) (-2.672074, 4.120524) (-2.674194, 4.122899) (-2.676376, 4.125323) (-2.678619, 4.127795) (-2.680924, 4.130313) (-2.683291, 4.132877) (-2.685719, 4.135485) (-2.688209, 4.138137) (-2.69076, 4.140832) (-2.693372, 4.143569) (-2.696046, 4.146347) (-2.698781, 4.149165) (-2.701577, 4.152023) (-2.704435, 4.154919) (-2.707354, 4.157854) (-2.710333, 4.160825) (-2.713374, 4.163832) (-2.716475, 4.166875) (-2.719637, 4.169953) (-2.72286, 4.173064) (-2.726144, 4.176209) (-2.729488, 4.179385) (-2.732893, 4.182594) (-2.736358, 4.185834) (-2.739884, 4.189103) (-2.74347, 4.192402) (-2.747116, 4.19573) (-2.750822, 4.199087) (-2.754588, 4.20247) (-2.758415, 4.20588) (-2.762301, 4.209317) (-2.766246, 4.212779) (-2.770252, 4.216265) (-2.774317, 4.219776) (-2.778442, 4.22331) (-2.782626, 4.226867) (-2.786869, 4.230446) (-2.791172, 4.234047) (-2.795533, 4.237669) (-2.799954, 4.241312) (-2.804434, 4.244974) (-2.808972, 4.248655) (-2.813569, 4.252355) (-2.818225, 4.256073) (-2.822939, 4.259809) (-2.827712, 4.263561) (-2.832543, 4.26733) (-2.837432, 4.271115) (-2.842379, 4.274915) (-2.847385, 4.278729) (-2.852448, 4.282558) (-2.857569, 4.286401) (-2.862747, 4.290256) (-2.867983, 4.294125) (-2.873277, 4.298005) (-2.878627, 4.301897) (-2.884035, 4.3058) (-2.8895, 4.309713) (-2.895022, 4.313637) (-2.900601, 4.31757) (-2.906237, 4.321513) (-2.911929, 4.325463) (-2.917678, 4.329422) (-2.923482, 4.333389) (-2.929344, 4.337363) (-2.935261, 4.341344) (-2.941234, 4.34533) (-2.947263, 4.349323) (-2.953348, 4.353321) (-2.959489, 4.357324) (-2.965685, 4.361331) (-2.971936, 4.365343) (-2.978243, 4.369358) (-2.984604, 4.373376) (-2.991021, 4.377397) (-2.997493, 4.38142) (-3.004019, 4.385445) (-3.0106, 4.389471) (-3.017235, 4.393499) (-3.023924, 4.397527) (-3.030668, 4.401555) (-3.037466, 4.405583) (-3.044318, 4.409611) (-3.051223, 4.413637) (-3.058182, 4.417663) (-3.065195, 4.421686) (-3.072261, 4.425707) (-3.07938, 4.429726) (-3.086552, 4.433742) (-3.093777, 4.437754) (-3.101056, 4.441763) (-3.108386, 4.445768) (-3.11577, 4.449768) (-3.123205, 4.453764) (-3.130693, 4.457754) (-3.138233, 4.461739) (-3.145825, 4.465718) (-3.153469, 4.469691) (-3.161164, 4.473657) (-3.168911, 4.477616) (-3.17671, 4.481568) (-3.184559, 4.485512) (-3.19246, 4.489449) (-3.200412, 4.493377) (-3.208415, 4.497297) (-3.216468, 4.501207) (-3.224571, 4.505108) (-3.232725, 4.509) (-3.24093, 4.512882) (-3.249184, 4.516753) (-3.257488, 4.520614) (-3.265842, 4.524464) (-3.274246, 4.528302) (-3.282699, 4.532129) (-3.291202, 4.535945) (-3.299753, 4.539748) (-3.308354, 4.543538) (-3.317004, 4.547316) (-3.325702, 4.551081) (-3.334449, 4.554832) (-3.343244, 4.55857) (-3.352087, 4.562294) (-3.360979, 4.566003) (-3.369918, 4.569698) (-3.378906, 4.573378) (-3.387941, 4.577043) (-3.397023, 4.580693) (-3.406153, 4.584327) (-3.41533, 4.587945) (-3.424554, 4.591546) (-3.433824, 4.595131) (-3.443142, 4.598699) (-3.452506, 4.602251) (-3.461916, 4.605784) (-3.471373, 4.609301) (-3.480876, 4.612799) (-3.490424, 4.616279) (-3.500019, 4.619741) (-3.509659, 4.623184) (-3.519344, 4.626608) (-3.529075, 4.630013) (-3.538851, 4.633399) (-3.548671, 4.636764) (-3.558537, 4.64011) (-3.568447, 4.643436) (-3.578402, 4.646741) (-3.588401, 4.650026) (-3.598444, 4.653289) (-3.608531, 4.656532) (-3.618662, 4.659752) (-3.628837, 4.662952) (-3.639055, 4.666129) (-3.649317, 4.669284) (-3.659621, 4.672417) (-3.669969, 4.675527) (-3.68036, 4.678615) (-3.690793, 4.681679) (-3.701269, 4.68472) (-3.711787, 4.687737) (-3.722347, 4.690731) (-3.732949, 4.693701) (-3.743594, 4.696647) (-3.75428, 4.699568) (-3.765007, 4.702464) (-3.775776, 4.705336) (-3.786586, 4.708182) (-3.797437, 4.711004) (-3.808329, 4.713799) (-3.819262, 4.716569) (-3.830235, 4.719314) (-3.841249, 4.722032) (-3.852302, 4.724723) (-3.863396, 4.727389) (-3.87453, 4.730027) (-3.885704, 4.732638) (-3.896917, 4.735223) (-3.908169, 4.73778) (-3.919461, 4.740309) (-3.930791, 4.742811) (-3.942161, 4.745285) (-3.953569, 4.74773) (-3.965016, 4.750148) (-3.976501, 4.752536) (-3.988024, 4.754896) (-3.999586, 4.757228) (-4.011185, 4.75953) (-4.022822, 4.761803) (-4.034497, 4.764046) (-4.046208, 4.76626) (-4.057958, 4.768444) (-4.069744, 4.770598) (-4.081567, 4.772721) (-4.093426, 4.774815) (-4.105322, 4.776878) (-4.117255, 4.77891) (-4.129223, 4.780911) (-4.141228, 4.782881) (-4.153268, 4.78482) (-4.165345, 4.786728) (-4.177456, 4.788604) (-4.189603, 4.790449) (-4.201786, 4.792261) (-4.214003, 4.794041) (-4.226254, 4.795789) (-4.238541, 4.797505) (-4.250862, 4.799187) (-4.263216, 4.800837) (-4.275606, 4.802455) (-4.288029, 4.804039) (-4.297995, 4.80528) (-4.305485, 4.806196) (-4.310485, 4.8068) (-4.312986, 4.807101) knots 0 0 0 0 0 0 0.00416667 0.00833333 0.0125 0.01666667 0.02083333 0.025 0.02916667 0.03333333 0.0375 0.04166667 0.04583333 0.05 0.05416667 0.05833333 0.0625 0.06666667 0.07083333 0.075 0.07916667 0.08333333 0.0875 0.09166667 0.09583333 0.1 0.10416667 0.10833333 0.1125 0.11666667 0.12083333 0.125 0.12916667 0.13333333 0.1375 0.14166667 0.14583333 0.15 0.15416667 0.15833333 0.1625 0.16666667 0.17083333 0.175 0.17916667 0.18333333 0.1875 0.19166667 0.19583333 0.2 0.20416667 0.20833333 0.2125 0.21666667 0.22083333 0.225 0.22916667 0.23333333 0.2375 0.24166667 0.24583333 0.25 0.25416667 0.25833333 0.2625 0.26666667 0.27083333 0.275 0.27916667 0.28333333 0.2875 0.29166667 0.29583333 0.3 0.30416667 0.30833333 0.3125 0.31666667 0.32083333 0.325 0.32916667 0.33333333 0.3375 0.34166667 0.34583333 0.35 0.35416667 0.35833333 0.3625 0.36666667 0.37083333 0.375 0.37916667 0.38333333 0.3875 0.39166667 0.39583333 0.4 0.40416667 0.40833333 0.4125 0.41666667 0.42083333 0.425 0.42916667 0.43333333 0.4375 0.44166667 0.44583333 0.45 0.45416667 0.45833333 0.4625 0.46666667 0.47083333 0.475 0.47916667 0.48333333 0.4875 0.49166667 0.49583333 0.5 0.50416667 0.50833333 0.5125 0.51666667 0.52083333 0.525 0.52916667 0.53333333 0.5375 0.54166667 0.54583333 0.55 0.55416667 0.55833333 0.5625 0.56666667 0.57083333 0.575 0.57916667 0.58333333 0.5875 0.59166667 0.59583333 0.6 0.60416667 0.60833333 0.6125 0.61666667 0.62083333 0.625 0.62916667 0.63333333 0.6375 0.64166667 0.64583333 0.65 0.65416667 0.65833333 0.6625 0.66666667 0.67083333 0.675 0.67916667 0.68333333 0.6875 0.69166667 0.69583333 0.7 0.70416667 0.70833333 0.7125 0.71666667 0.72083333 0.725 0.72916667 0.73333333 0.7375 0.74166667 0.74583333 0.75 0.75416667 0.75833333 0.7625 0.76666667 0.77083333 0.775 0.77916667 0.78333333 0.7875 0.79166667 0.79583333 0.8 0.80416667 0.80833333 0.8125 0.81666667 0.82083333 0.825 0.82916667 0.83333333 0.8375 0.84166667 0.84583333 0.85 0.85416667 0.85833333 0.8625 0.86666667 0.87083333 0.875 0.87916667 0.88333333 0.8875 0.89166667 0.89583333 0.9 0.90416667 0.90833333 0.9125 0.91666667 0.92083333 0.925 0.92916667 0.93333333 0.9375 0.94166667 0.94583333 0.95 0.95416667 0.95833333 0.9625 0.96666667 0.97083333 0.975 0.97916667 0.98333333 0.9875 0.99166667 0.99583333 1 1 1 1 1 1
  arc A15 (-4.312986, 4.807101) -> (-4.807101, 4.312986) centre (0, 0) ccw